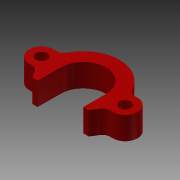
# Autodesk Inventor part: plastic_part_13
Saved by Autodesk Inventor 2013 (Build 170138000, 138)
## iProperties
Shininess: 20.0
Created: 2014-03-04
Part Number: plastic_part_13
Document SubType Name: Modeling
Designer: Noa Izumi
Material: Default
Density: 1 g/cm^3
Density: 0.0
Volumn: 0.0
Area: 0.0
PropertySet Name: Model Information
Control State: 0
Master: False
Checked Out: False
Author: Noa Izumi
Autodesk Inventor part; units mm, degrees
ref_plane "YZ Plane" through (0, 0, 0) normal (1, 0, 0) x (0, 1, 0)
ref_plane "XZ Plane" through (0, 0, 0) normal (0, 1, 0) x (-1, 0, 0)
ref_plane "XY Plane" through (0, 0, 0) normal (0, 0, 1) x (1, 0, 0)
sketch "Sketch1" plane through (0, 0, 0) normal (0, 0, 1) x (1, 0, 0)
  circle A0 centre (0, 0) radius 9.5
  circle A1 centre (-11, 0) radius 3.25
  circle A2 centre (11, 0) radius 3.25
  line L0 (-11, 3.25) -> (11, 3.25)
  line L1 (11, 3.25) -> (11, -3.25)
  line L2 (11, -3.25) -> (-11, -3.25)
  line L3 (-11, -3.25) -> (-11, 3.25)
  dimension "d15" = 6.5
  dimension "d17" = 6.5
  dimension "d12" = 19
  dimension "d16" = 11
  dimension "d18" = 11
  constraints: 8 end point, 2 parallel, 2 vertical alignment, 1 centre point, 1 horizontal, 1 perpendicular, 4 other
  measures "d12" diameter of A0
  measures "d16" distance of point (-11, 0) A0.centre
  measures "d18" distance of point (11, 0) A0.centre
extrude "Extrusion1" add sketch "Sketch1" along normal blind 6
sketch "草圖4" plane through (0, 0, 6) normal (0, 0, 1) x (1, 0, 0)
  arc A0 (-8.9268, -3.25) -> (8.9268, -3.25) centre (0, 0) ccw projected
  circle A1 centre (0, 0) radius 6
  line L0 (-6, 0) -> (6, 0)
  line L1 (6, 0) -> (6, -9.5)
  line L2 (6, -9.5) -> (-6, -9.5)
  line L3 (-6, -9.5) -> (-6, 0)
  line L4 (-8, -9.5) -> (8, -9.5)
  line L5 (8, -9.5) -> (8, -6)
  line L6 (8, -6) -> (-8, -6)
  line L7 (-8, -6) -> (-8, -9.5)
  dimension "d19" = 12
  dimension "d23" = 6
  dimension "d24" = 3.5
  dimension "d26" = 16
  dimension "d27" = 8
  constraints: 16 end point, 4 parallel, 2 horizontal, 2 perpendicular, 1 coincident, 1 horizontal alignment, 2 other
  measures "d23" distance between parallel lines of L6 L0
  measures "d24" distance of L4.end L5.end
  measures "d26" distance of L4.start L4.end
  measures "d27" distance from line of A0.centre L7
extrude "擠出2" cut sketch "草圖4" against normal through all
fillet "圓角2" radius 2 4 edges at (8.9268, -3.25, 3) (-8.9268, -3.25, 3) (8.9268, 3.25, 3) (-8.9268, 3.25, 3)
sketch "草圖5" plane through (0, 0, 6) normal (0, 0, 1) x (1, 0, 0)
  arc A0 (14.25, 0) -> (11, 3.25) centre (11, 0) ccw projected
  arc A1 (-11, 3.25) -> (-11, -3.25) centre (-11, 0) ccw projected
  constraints: 2 coincident
hole "孔2" at (-11, 0, 6) at (11, 0, 6) direction (0, 0, -1) diameter 3 end through all
